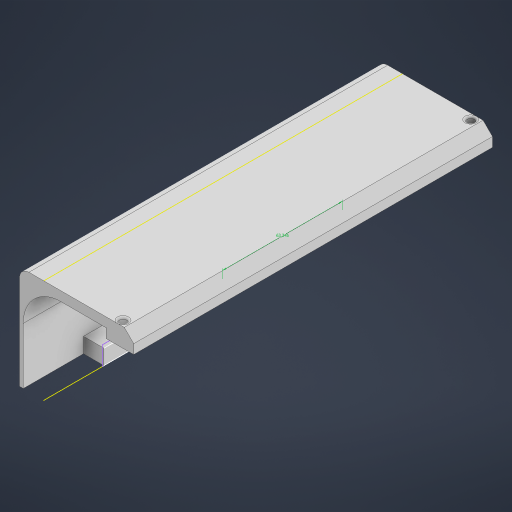
# Autodesk Inventor part: bumper belakang
Saved by Autodesk Inventor 2024.3 (Build 283343000, 343)
## iProperties
Created: 2025-06-14
Part Number: bumper belakang
Material: Generic
Document SubType Name: Modeling
Designer: Akbar Syihabuddin
Density: 1 g/cm^3
Appearance: Default
Author: Akbar Syihabuddin
Autodesk Inventor part; units mm, degrees
ref_plane "YZ Plane" through (0, 0, 0) normal (1, 0, 0) x (0, 1, 0)
ref_plane "XZ Plane" through (0, 0, 0) normal (0, 1, 0) x (-1, 0, 0)
ref_plane "XY Plane" through (0, 0, 0) normal (0, 0, 1) x (1, 0, 0)
sketch "Sketch1" plane through (0, 0, 0) normal (0, 1, 0) x (-1, 0, 0)
  line L0 (-32.3469, 68.4305) -> (-32.3469, -55.5695)
  line L1 (-17.6425, -88.9147) -> (-32.3469, -88.9147)
  line L2 (-32.3469, -88.9147) -> (-32.3469, -55.5695)
  line L3 (-32.3469, -55.5695) -> (-17.6425, -55.5695)
  line L4 (-17.6425, -55.5695) -> (-17.6425, -88.9147)
  line L5 (-27.3469, -55.5695) -> (-27.3469, 68.4305)
  line L6 (-32.3469, -55.5695) -> (-27.3469, -55.5695)
  line L7 (-27.3469, -55.5695) -> (-27.3469, 68.4305)
  line L8 (-27.3469, 68.4305) -> (-32.3469, 68.4305)
  line L9 (-32.3469, 68.4305) -> (-32.3469, -55.5695)
  line L10 (-32.3469, 68.4305) -> (-17.6425, 68.4305)
  line L11 (-17.6425, 68.4305) -> (-17.6425, 101.7757)
  line L12 (-17.6425, 101.7757) -> (-32.3469, 101.7757)
  line L13 (-32.3469, 101.7757) -> (-32.3469, 68.4305)
  point P0 (0, 0)
  point P1 (25.2053, -93.5695)
  constraints: 28 end point, 6 parallel, 3 horizontal, 3 perpendicular
extrude "Extrusion1" add sketch "Sketch1" along normal blind 10
chamfer "Chamfer1" distance 5 angle 45 1 edges at (32.3469, 10, 6.4305)
sketch "Sketch2" plane through (17.6425, 0, -88.9147) normal (-1, 0, 0) x (0, 0, 1)
  line L0 (0, 0) -> (0, 10) projected
  line L1 (33.3452, 0) -> (33.3452, 10) projected
  line L2 (0, 10) -> (33.3452, 10)
  line L3 (33.3452, 10) -> (33.3452, 5)
  line L4 (33.3452, 5) -> (0, 5)
  line L5 (0, 5) -> (0, 10)
  line L6 (157.3452, 10) -> (190.6905, 10) projected
  line L7 (157.3452, 0) -> (157.3452, 10) projected
  line L8 (190.6905, 10) -> (157.3452, 10)
  line L9 (157.3452, 10) -> (157.3452, 5)
  line L10 (157.3452, 5) -> (190.6905, 5)
  line L11 (190.6905, 5) -> (190.6905, 10)
  point P0 (88.9147, 0)
  dimension "d5" = 5
  constraints: 16 end point, 4 parallel, 2 horizontal, 2 midpoint, 2 perpendicular
  measures "d5" distance of L2.end L3.end
extrude "Extrusion2" add sketch "Sketch2" along normal blind 46
sketch "Sketch3" plane through (17.6425, 5, -88.9147) normal (0, -1, 0) x (1, 0, 0)
  line L0 (9.7044, 0) -> (-46, 0) projected
  line L1 (9.7044, 33.3452) -> (-46, 33.3452) projected
  line L2 (-46, 0) -> (-44, 0)
  line L3 (-44, 0) -> (-44, 33.3452)
  line L4 (-44, 33.3452) -> (-46, 33.3452)
  line L5 (-46, 33.3452) -> (-46, 0)
  line L6 (9.7044, 190.6905) -> (-46, 190.6905) projected
  line L7 (9.7044, 157.3452) -> (-46, 157.3452) projected
  line L8 (-46, 190.6905) -> (-45, 190.6905)
  line L9 (-45, 190.6905) -> (-45, 157.3452)
  line L10 (-45, 157.3452) -> (-46, 157.3452)
  line L11 (-46, 157.3452) -> (-46, 190.6905)
  point P0 (-17.6425, 88.9147)
  dimension "d8" = 2
  constraints: 16 end point, 4 parallel, 2 horizontal, 2 perpendicular, 2 point on line
  measures "d8" distance of L4.end L3.end
extrude "Extrusion3" add sketch "Sketch3" along normal blind 45
sketch "Sketch4" plane through (27.3469, 0, 68.4305) normal (0, 0, -1) x (-1, 0, 0)
  line L0 (0, 10) -> (55.7044, 10) projected
  line L1 (0, 0) -> (9.7517, 0)
  line L2 (9.7517, 0) -> (9.7517, 10)
  line L3 (9.7517, 10) -> (0, 10)
  line L4 (0, 10) -> (0, 0)
  line L5 (9.7517, 5) -> (55.7044, 5)
  line L6 (55.7044, 5) -> (55.7044, 10)
  line L7 (55.7044, 10) -> (9.7517, 10)
  line L8 (9.7517, 10) -> (9.7517, 5)
  line L9 (54.7044, 5) -> (54.7044, -40) projected
  line L10 (55.7044, 5) -> (54.7044, 5)
  line L11 (54.7044, 5) -> (54.7044, -40)
  line L12 (54.7044, -40) -> (55.7044, -40)
  line L13 (55.7044, -40) -> (55.7044, 5)
  point P0 (27.3469, 0)
  constraints: 24 end point, 6 parallel, 3 horizontal, 3 perpendicular, 1 midpoint, 1 point on line
extrude "Extrusion4" add sketch "Sketch4" along normal blind 150
sketch "Sketch5" plane through (-27.3575, 5, 101.7757) normal (1, 0, 0) x (0, 0, -1)
  line L0 (0, 0) -> (157.3452, 0) projected
  line L1 (190.6905, -45) -> (157.3452, -45) projected
  line L2 (0, 0) -> (157.3452, 0)
  line L3 (157.3452, 0) -> (157.3452, -45)
  line L4 (157.3452, -45) -> (0, -45)
  line L5 (0, -45) -> (0, 0)
  point P0 (101.7757, -5)
  constraints: 8 end point, 2 parallel, 1 horizontal, 1 perpendicular
extrude "Extrusion5" add sketch "Sketch5" along normal blind 1
sketch "Sketch8" plane through (17.6425, -40, -88.9147) normal (0, -1, 0) x (1, 0, 0)
  line L0 (-44, 0) -> (-44, 190.6905) projected
  line L1 (9.7044, 0) -> (-46, 0) projected
  line L2 (-44, 190.6905) -> (-46, 190.6905)
  line L3 (-46, 190.6905) -> (-46, 0)
  line L4 (-46, 0) -> (-44, 0)
  line L5 (-44, 0) -> (-44, 190.6905)
  point P0 (-17.6425, 88.9147)
  constraints: 8 end point, 2 parallel, 1 horizontal, 1 perpendicular
extrude "Extrusion8" add sketch "Sketch8" along normal blind 5
sketch "Sketch9" plane through (-26.3575, 5, 101.7757) normal (1, 0, 0) x (0, 0, -1)
  line L0 (0, 0) -> (0, -50) projected
  line L1 (0, -50) -> (32, -50)
  line L2 (0, -50) -> (190.6905, -50) projected
  line L3 (190.6905, -50) -> (158.6905, -50)
  line L4 (32, -50) -> (155.0848, -50)
  line L5 (155.0848, -50) -> (155.0848, -42)
  line L6 (155.0848, -42) -> (32, -42)
  line L7 (32, -42) -> (32, -50)
  point P0 (101.7757, -5)
  dimension "d29" = 32
  dimension "d30" = 32
  dimension "d31" = 8
  constraints: 12 end point, 2 parallel, 2 point on line, 1 horizontal, 1 perpendicular
  measures "d29" distance of L0.end L1.end
  measures "d30" distance of L2.end L3.end
  measures "d31" distance of L5.end L4.end
extrude "Extrusion9" add sketch "Sketch9" along normal blind 10.786
sketch "Sketch10" plane through (-15.5715, 5, 101.7757) normal (1, 0, 0) x (0, 0, -1)
  line L0 (190.6905, 5) -> (0, 5) projected
  line L1 (95.3452, 5) -> (95.3452, -50)
  line L2 (0, -50) -> (190.6905, -50) projected
  circle A0 centre (49.4524, -47.1745) radius 1.5
  circle A1 centre (49.4524, -47.1745) radius 1.5
  circle A2 centre (79.4524, -47.1745) radius 1.5
  circle A3 centre (79.4524, -47.1745) radius 1.5
  circle A4 centre (109.4524, -47.1745) radius 1.5
  circle A5 centre (109.4524, -47.1745) radius 1.5
  circle A6 centre (139.4524, -47.1745) radius 1.5
  circle A7 centre (139.4524, -47.1745) radius 1.5
  line L3 (157.7974, -50) -> (157.7974, -40)
  line L4 (31.1074, -40) -> (31.1074, -50)
  line L5 (31.1074, -40) -> (157.7974, -40)
  line L6 (157.7974, -40) -> (157.7974, -50)
  line L7 (157.7974, -50) -> (31.1074, -50)
  line L8 (31.1074, -50) -> (31.1074, -40)
  line L9 (95.3452, -50) -> (95.3452, -40)
  line L10 (155.0848, -42) -> (32, -42) projected
  line L11 (95.3452, -42) -> (32, -42)
  line L12 (95.3452, -42) -> (158.6902, -42)
  line L13 (158.6902, -42) -> (158.6902, -50)
  line L14 (158.6902, -50) -> (155.0848, -50)
  line L15 (155.0848, -50) -> (155.0848, -42) projected
  line L16 (155.0848, -50) -> (155.0848, -42)
  line L17 (155.0848, -42) -> (158.6902, -42)
  point P0 (101.7757, -5)
  point P1 (155.0848, -50)
  dimension "d34" = 63.345
  constraints: 28 end point, 8 centre point, 7 point on line, 4 coincident, 3 perpendicular, 2 collinear, 2 midpoint, 2 parallel, 1 horizontal, 1 vertical
  measures "d34" distance of L11.start L12.end
extrude "Extrusion10" add sketch "Sketch10" against normal blind 10.786 contours L12 L3 L2 L15 | L12 L13 L2 L3
fillet "Fillet1" radius 5 1 edges at (-28.3575, 10, 6.4305)
fillet "Fillet2" radius 20 1 edges at (-26.3575, 5, 6.4305)
fillet "Fillet4" radius 4 1 edges at (17.5953, 5, -6.5695)
sketch "Sketch11" plane through (0, 10, 0) normal (0, 1, 0) x (1, 0, 0)
  circle A0 centre (23.7073, 85.9487) radius 2
  circle A1 centre (23.7073, 85.9487) radius 1.5
  line L0 (32.3469, -101.7757) -> (32.3469, 88.9147) projected
  line L1 (32.3469, -6.4305) -> (-25.9991, -6.4305)
  circle A2 centre (23.7073, -98.8097) radius 2
  circle A3 centre (23.7073, -98.8097) radius 1.5
  point P0 (0, 0)
  dimension "d43" = 4
  dimension "d44" = 3
  constraints: 4 centre point, 2 coincident, 2 end point, 2 symmetric about line, 1 horizontal, 1 midpoint, 2 other
  measures "d43" diameter of A0
  measures "d44" diameter of A1
extrude "Extrusion12" cut sketch "Sketch11" against normal blind 4 contours A0 | A1 | A2 | A3
extrude "Extrusion13" cut sketch "Sketch11" against normal blind 100 contours A1 | A3
fillet "Fillet5" radius 1 1 edges at (21.7073, 10, -85.9487)
fillet "Fillet6" radius 1 1 edges at (21.7073, 10, 98.8097)
sketch "Sketch12" plane through (-15.5715, 5, 101.7757) normal (1, 0, 0) x (0, 0, -1)
  line L0 (33.3452, -5) -> (157.3452, -5)
  line L1 (95.3452, -5) -> (95.3452, -50)
  line L2 (94.0723, -38) -> (94.0723, -50)
  line L3 (33.5543, -44.5) -> (157.1905, -44.5)
  circle A0 centre (104.2097, -44.5) radius 1.4
  circle A1 centre (129.8962, -44.5) radius 1.4
  circle A2 centre (86.4808, -44.5) radius 1.4
  circle A3 centre (60.7943, -44.5) radius 1.4
  line L4 (32.0002, -40) -> (158.6902, -40)
  line L5 (158.6902, -50) -> (158.6902, -40)
  line L6 (32.0002, -40) -> (158.6902, -40)
  line L7 (158.6902, -40) -> (158.6902, -50)
  line L8 (158.6902, -50) -> (32.0002, -50)
  line L9 (32.0002, -50) -> (32.0002, -40)
  point P0 (101.7757, -5)
  point P1 (13.9577, -136.3434)
  dimension "d52" = 2.8
  dimension "d53" = 2.8
  constraints: 20 end point, 4 centre point, 3 parallel, 2 symmetric about line, 1 horizontal, 1 midpoint, 1 perpendicular, 1 point on line, 2 other
  measures "d52" diameter of A0
  measures "d53" diameter of A1
extrude "Extrusion14" cut sketch "Sketch12" against normal blind 100 contours A1 L3 | L3 A1 | A0 L3 | L3 A0 | A3 L3 | L3 A3 | A2 L3 | L3 A2
body "Solid1"
